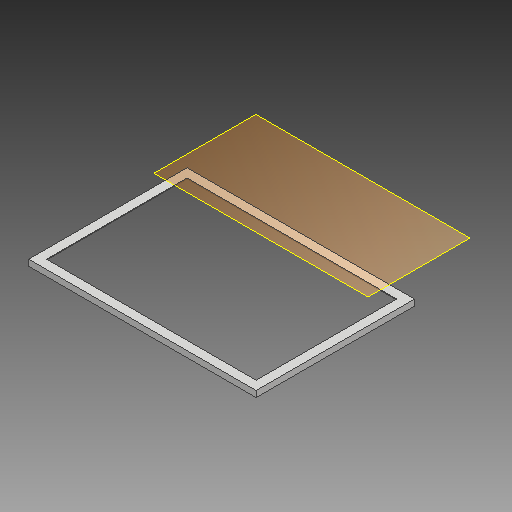
# Autodesk Inventor part: DummyAuschnitt
Saved by Autodesk Inventor 2017 (Build 210142000, 142)
## iProperties
Part Number: DummyAuschnitt
Material: Generisch
Document SubType Name: Modeling
Designer: aXe
Density: 1 g/cm^3
Appearance: Vorgabe
Author: aXe
Autodesk Inventor part; units mm, degrees
ref_plane "YZ Plane" through (0, 0, 0) normal (1, 0, 0) x (0, 1, 0)
ref_plane "Arbeitsebene1" through (-8.2728, 45.0264, 0) normal (0, 0, 1) x (1, 0, 0)
sketch "Skizze1" plane through (-8.2728, 45.0264, 0) normal (0, 0, 1) x (1, 0, 0)
  line L0 (55.3228, -80.3764) -> (55.3228, -17.2764) projected
  line L1 (55.3228, -17.2764) -> (-38.7772, -17.2764) projected
  line L2 (-38.7772, -17.2764) -> (-38.7772, -80.3764) projected
  line L3 (-38.7772, -80.3764) -> (55.3228, -80.3764) projected
  line L4 (-38.7772, -17.2764) -> (-38.8772, -17.2764)
  line L5 (-38.8772, -17.2764) -> (-38.8772, -17.1764)
  line L6 (-38.8772, -17.1764) -> (-38.7772, -17.1764)
  line L7 (-38.7772, -17.1764) -> (-38.7772, -17.2764)
  line L8 (55.3228, -80.3764) -> (55.4228, -80.3764)
  line L9 (55.4228, -80.3764) -> (55.4228, -80.4764)
  line L10 (55.4228, -80.4764) -> (55.3228, -80.4764)
  line L11 (55.3228, -80.4764) -> (55.3228, -80.3764)
  line L12 (-38.8772, -17.1764) -> (55.4228, -17.1764)
  line L13 (55.4228, -17.1764) -> (55.4228, -80.4764)
  line L14 (55.4228, -80.4764) -> (-38.8772, -80.4764)
  line L15 (-38.8772, -80.4764) -> (-38.8772, -17.1764)
  point P0 (8.2728, -45.0264)
  dimension "d0" = 0.1
  dimension "d1" = 0.1
  dimension "d2" = 0.1
  dimension "d3" = 0.1
  constraints: 24 end point, 6 parallel, 3 horizontal, 3 perpendicular
  measures "d0" distance of L5.end L6.end
  measures "d1" distance of L4.end L5.end
  measures "d2" distance of L9.end L10.end
  measures "d3" distance of L8.end L9.end
ref_plane "Arbeitsebene2" through (-47.05, -35.35, -2.75) normal (0, 0, -1) x (0, 1, 0)
ref_plane "Arbeitsebene3" through (-8.2728, 45.0264, 0) normal (0, 0, 1) x (1, 0, 0)
ref_plane "Arbeitsebene4" through (-47.05, -35.35, -2.75) normal (0, 0, -1) x (0, 1, 0)
sketch "Skizze2" plane through (-8.2728, 45.0264, 0) normal (0, 0, 1) x (1, 0, 0)
  line L0 (55.3228, -80.3764) -> (55.3228, -17.2764) projected
  line L1 (55.3228, -17.2764) -> (-38.7772, -17.2764) projected
  line L2 (-38.7772, -17.2764) -> (-38.7772, -80.3764) projected
  line L3 (-38.7772, -80.3764) -> (55.3228, -80.3764) projected
  line L4 (-38.7772, -17.2764) -> (-42.7772, -17.2764)
  line L5 (-42.7772, -17.2764) -> (-42.7772, -13.2764)
  line L6 (-42.7772, -13.2764) -> (-38.7772, -13.2764)
  line L7 (-38.7772, -13.2764) -> (-38.7772, -17.2764)
  line L8 (55.3228, -80.3764) -> (59.3228, -80.3764)
  line L9 (59.3228, -80.3764) -> (59.3228, -84.3764)
  line L10 (59.3228, -84.3764) -> (55.3228, -84.3764)
  line L11 (55.3228, -84.3764) -> (55.3228, -80.3764)
  line L12 (-42.7772, -13.2764) -> (59.3228, -13.2764)
  line L13 (59.3228, -13.2764) -> (59.3228, -84.3764)
  line L14 (59.3228, -84.3764) -> (-42.7772, -84.3764)
  line L15 (-42.7772, -84.3764) -> (-42.7772, -13.2764)
  point P0 (8.2728, -45.0264)
  dimension "d6" = 4
  dimension "d7" = 4
  dimension "d8" = 4
  dimension "d9" = 4
  constraints: 24 end point, 6 parallel, 3 horizontal, 3 perpendicular
  measures "d6" distance of L5.end L6.end
  measures "d7" distance of L4.end L5.end
  measures "d8" distance of L9.end L10.end
  measures "d9" distance of L8.end L9.end
extrude "Extrusion2" add sketch "Skizze2" against normal up to surface (2.75 mm away)
extrude "Extrusion3" cut sketch "Skizze1" against normal up to surface (2.75 mm away) contours L3 L2 L1 L0
chamfer "Fase1" distance 2.4 angle 45 4 edges at (0, -35.35, -2.75) (-47.05, -3.8, -2.75) (47.05, -3.8, -2.75) (0, 27.75, -2.75)
